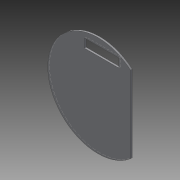
# Autodesk Inventor part: Mid Plate
Saved by Autodesk Inventor 2015 (Build 190159000, 159)
## iProperties
Created: 2014-07-28
Part Number: Mid Plate
Material: Generic
Document SubType Name: Modeling
Designer: karl
Density: 1 g/cm^3
Appearance: Default
Author: karl
Autodesk Inventor part; units mm, degrees
ref_plane "YZ Plane" through (0, 0, 0) normal (1, 0, 0) x (0, 1, 0)
ref_plane "XZ Plane" through (0, 0, 0) normal (0, 1, 0) x (-1, 0, 0)
ref_plane "XY Plane" through (0, 0, 0) normal (0, 0, 1) x (1, 0, 0)
sketch "Sketch1" plane through (0, 0, 0) normal (0, 1, 0) x (-1, 0, 0)
  circle A0 centre (0, 0) radius 85
  line L0 (-55, 64.8074) -> (-55, -64.8074)
  line L1 (23, 75) -> (-35, 75)
  line L2 (-35, 75) -> (-35, 60)
  line L3 (-35, 60) -> (23, 60)
  line L4 (23, 60) -> (23, 75)
  line L5 (-6, 60) -> (-6, 30.4166)
  line L6 (23, -60) -> (-35, -60)
  line L7 (-35, -60) -> (-35, -75)
  line L8 (-35, -75) -> (23, -75)
  line L9 (23, -75) -> (23, -60)
  dimension "d0" = 170
  dimension "d1" = 55
  dimension "d2" = 58
  dimension "d3" = 15
  dimension "d4" = 49
  dimension "d5" = 60
  dimension "d8" = 60
  constraints: 20 end point, 4 parallel, 3 collinear, 2 horizontal, 2 perpendicular, 2 point on circle, 2 vertical, 1 centre point, 1 coincident, 1 midpoint
  measures "d0" diameter of A0
  measures "d1" distance from line of point (0, 0) L0
  measures "d2" distance of L3.end L2.end
  measures "d3" distance of L1.end L2.end
  measures "d4" distance between parallel lines of L0 L5
  measures "d5" distance from line of point (0, 0) L3
  measures "d8" distance from line of L6 point (0, 0)
extrude "Extrusion1" add sketch "Sketch1" along normal blind 3 contours A0 L0 picked at (43.6667, 0)
sketch "Sketch2" plane through (0, 0, 0) normal (0, -1, 0) x (1, 0, 0)
  line L0 (-23, 60) -> (-13, 60)
  line L1 (-13, 60) -> (-13, 57)
  line L2 (-13, 57) -> (-23, 57)
  line L3 (-23, 57) -> (-23, 60)
  line L4 (35, 60) -> (25, 60)
  line L5 (25, 60) -> (25, 57)
  line L6 (25, 57) -> (35, 57)
  line L7 (35, 57) -> (35, 60)
  point P0 (0, 0)
  dimension "d9" = 10
  dimension "d10" = 3
  dimension "d11" = 10
  dimension "d12" = 3
  constraints: 16 end point, 4 parallel, 2 horizontal, 2 perpendicular
  measures "d9" distance of L1.end L2.end
  measures "d10" distance of L0.end L1.end
  measures "d11" distance of L6.end L5.end
  measures "d12" distance of L5.end L4.end
extrude "Extrusion2" cut sketch "Sketch2" against normal blind 3
sketch "Sketch3" plane through (0, 0, 0) normal (0, -1, 0) x (1, 0, 0)
  line L0 (18.5, 37) -> (21.5, 37)
  line L1 (21.5, 37) -> (21.5, 27)
  line L2 (21.5, 27) -> (18.5, 27)
  line L3 (18.5, 27) -> (18.5, 37)
  line L4 (35, 57) -> (25, 57) projected
  line L5 (-13, 60) -> (25, 60) construction
  line L6 (6, 60) -> (6, 41.1412) construction
  point P0 (0, 0)
  dimension "d15" = 3
  dimension "d16" = 10
  dimension "d17" = 20
  dimension "d18" = 12.5
  constraints: 10 end point, 2 parallel, 1 horizontal, 1 midpoint, 1 perpendicular, 1 vertical
  measures "d15" distance of L1.end L2.end
  measures "d16" distance of L0.end L1.end
  measures "d17" distance between parallel lines of L4 L0
  measures "d18" distance between parallel lines of L3 L6
extrude "Extrusion3" cut sketch "Sketch3" against normal blind 3
sketch "Sketch4" plane through (0, 0, 0) normal (0, -1, 0) x (1, 0, 0)
  line L0 (-69.5, 30) -> (-66.5, 30)
  line L1 (-66.5, 30) -> (-66.5, 20)
  line L2 (-66.5, 20) -> (-69.5, 20)
  line L3 (-69.5, 20) -> (-69.5, 30)
  line L4 (55, 64.8074) -> (55, -64.8074) projected
  line L5 (-69.5, 5) -> (-66.5, 5)
  line L6 (-66.5, 5) -> (-66.5, -5)
  line L7 (-66.5, -5) -> (-69.5, -5)
  line L8 (-69.5, -5) -> (-69.5, 5)
  point P0 (0, 0)
  point P1 (-69.5, 0)
  dimension "d21" = 3
  dimension "d22" = 10
  dimension "d23" = 124.5
  dimension "d24" = 30
  dimension "d25" = 3
  dimension "d26" = 10
  constraints: 16 end point, 4 parallel, 2 horizontal, 2 perpendicular, 1 collinear, 1 horizontal alignment, 1 midpoint
  measures "d21" distance of L1.end L2.end
  measures "d22" distance of L0.end L1.end
  measures "d23" distance between parallel lines of L4 L3
  measures "d24" distance from line of point (0, 0) L0
  measures "d25" distance of L6.end L7.end
  measures "d26" distance of L5.end L6.end
extrude "Extrusion4" cut sketch "Sketch4" against normal blind 3
mirror "Mirror1" about plane through (0, 0, 0) normal (0, 0, 1) of "Extrusion3", "Extrusion2", "Extrusion4"
sketch "Sketch5" plane through (0, 0, 0) normal (0, -1, 0) x (1, 0, 0)
  point P0 (0, 0)
equation "\"d8\" = d5"
body "Solid1"
